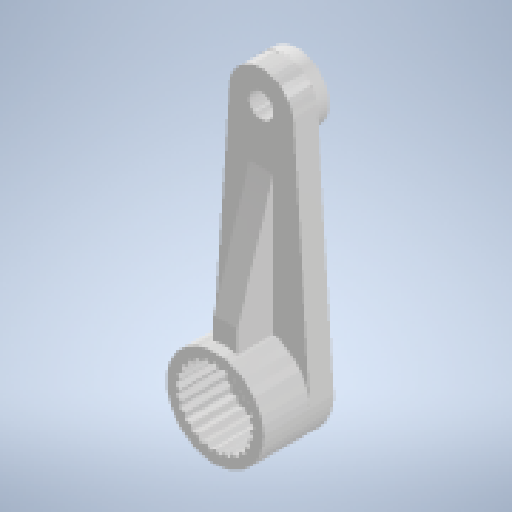
# Autodesk Inventor part: servo_arm_20131227-19207-m9y6rr-0
Saved by Autodesk Inventor 2024.2 (Build 282272000, 272)
## iProperties
Created: 2026-01-28
Part Number: servo_arm_20131227-19207-m9y6rr-0
Material: Типовые
Document SubType Name: Modeling
Designer: katya_notebook
Density: 1 g/cm^3
Appearance: По умолчанию
Author: katya_notebook
Autodesk Inventor part; units mm, degrees
ref_plane "YZ Plane" through (0, 0, 0) normal (1, 0, 0) x (0, 1, 0)
ref_plane "XZ Plane" through (0, 0, 0) normal (0, 1, 0) x (-1, 0, 0)
ref_plane "XY Plane" through (0, 0, 0) normal (0, 0, 1) x (1, 0, 0)
sketch "Эскиз1" plane through (2.707, 20, -6) normal (0, 0, -1) x (-1, 0, 0)
  circle A0 centre (2.7053, 0.0036) radius 2.7027 projected
  circle A1 centre (2.707, 0) radius 1 projected
  point P0 (2.707, -20)
extrude "Выдавливание1" add sketch "Эскиз1" along normal blind 1
